Autodesk Fusion 360 part; units mm, degrees
note: some values were not read from the file. Chosen so that the rebuilt part matches the saved one: which bodies a step acts on; which face or edge a step refers to. Set by a fixed rule: which sketch regions a step uses.
(part 2 of 2)
sketch "hookLedge" plane through (0, 0, -2.5) normal (0, 0, -1) x (1, 0, 0)
  circle A0 centre (54.2689, -22.0155) radius 1.5
  circle A1 centre (176.25, -22.3937) radius 1.5
  circle A2 centre (176, -22.3937) radius 1.25
  circle A3 centre (146, -22.3937) radius 1.25
  circle A4 centre (176, -22.3937) radius 1.25
  circle A5 centre (146, -22.3937) radius 1.25
  circle A6 centre (4, -22.3937) radius 1.25
  circle A7 centre (54, -22.3937) radius 1.25
  circle A8 centre (4, -22.3937) radius 1.25
  circle A9 centre (54, -22.3937) radius 1.25
  line L0 (0, 0) -> (0, -40)
  line L1 (0, -40) -> (180, -40)
  line L2 (180, -40) -> (180, 0)
  line L3 (180, 0) -> (0, 0)
  line L4 (140.5, -33.5) -> (140.5, -27.75)
  line L5 (140.5, -27.75) -> (148, -27.75)
  line L6 (154.5, -33.5) -> (154.5, -24.7385)
  line L7 (154.5, -24.7385) -> (120, -24.7385)
  line L8 (120, -24.7385) -> (120, -27.7385)
  line L9 (120, -27.7385) -> (116.5, -27.7385)
  line L10 (116.5, -27.7385) -> (116.5, -24.7385)
  line L11 (116.5, -24.7385) -> (25.5, -24.7385)
  line L12 (25.5, -24.7385) -> (25.5, -33.5)
  line L13 (32, -27.75) -> (39.5, -27.75)
  line L14 (39.5, -27.75) -> (39.5, -33.5)
  line L15 (25.5, -33.5) -> (32, -33.5)
  line L16 (50.5, -33.5) -> (50.5, -36.5)
  line L17 (50.5, -36.5) -> (2, -36.5)
  line L18 (2, -36.5) -> (2, -3.5)
  line L19 (2, -3.5) -> (50.5, -3.5)
  line L20 (50.5, -3.5) -> (50.5, -6.5)
  line L21 (50.5, -6.5) -> (35.5, -6.5)
  line L22 (35.5, -15.2615) -> (116.5, -15.2615)
  line L23 (116.5, -15.2615) -> (116.5, -12.2615)
  line L24 (116.5, -12.2615) -> (120, -12.2615)
  line L25 (120, -12.2615) -> (120, -15.2615)
  line L26 (120, -15.2615) -> (144.5, -15.2615)
  line L27 (144.5, -6.5) -> (129.5, -6.5)
  line L28 (129.5, -6.5) -> (129.5, -3.5)
  line L29 (129.5, -3.5) -> (178, -3.5)
  line L30 (178, -3.5) -> (178, -36.5)
  line L31 (178, -36.5) -> (129.5, -36.5)
  line L32 (129.5, -36.5) -> (129.5, -33.5)
  line L33 (129.5, -33.5) -> (140.5, -33.5)
  line L34 (25.5, -24.4885) -> (174.5, -24.4885)
  line L35 (32.5, -15.5115) -> (25.5, -15.5115)
  line L36 (100, -24.4885) -> (100.0375, -15.4143)
  line L37 (90, -40) -> (90, 0)
  circle A10 centre (145.75, -22.3937) radius 1.5
  circle A11 centre (3.75, -22.3937) radius 1.5
  line L38 (144.5, -15.2615) -> (144.5, -6.5)
  line L39 (148, -27.75) -> (148, -33.5)
  line L40 (32, -33.5) -> (32, -27.75)
  circle A12 centre (145.75, -22.3937) radius 1.5
  circle A13 centre (54.2765, -21.879) radius 1.5
  line L41 (25.5, -15.5115) -> (25.5, -24.4885)
  line L42 (34.75, -17.7615) -> (32.5, -15.5115)
  line L43 (174.5, -24.4885) -> (174.5, -15.5115)
  line L44 (174.5, -15.5115) -> (167.5, -15.5115)
  line L45 (167.5, -15.5115) -> (165.25, -17.7615)
  line L46 (165.25, -17.7615) -> (144, -17.7615)
  line L47 (144, -17.7615) -> (144, -15.5115)
  line L48 (56, -15.5115) -> (56, -17.7615)
  line L49 (56, -17.7615) -> (34.75, -17.7615)
  line L50 (148, -33.5) -> (154.5, -33.5)
  line L51 (39.5, -33.5) -> (50.5, -33.5)
  line L52 (35.5, -6.5) -> (35.5, -15.2615)
  line L53 (144, -15.5115) -> (56, -15.5115)
  point P0 (176.25, -22.3937)
  dimension "d122" = 3
  dimension "d123" = 3
  constraint midpoint L34 L36.start
  constraint midpoint L1 L37.start
  constraint midpoint L3 L37.end
  constraint symmetric A0 L36 A10
  constraint symmetric A1 L37 A11
  constraint coincident A10.centre A12.centre
  constraint coincident P0 A1.centre
  measures "d122" diameter of A0
  measures "d123" diameter of A1
extrude "Extrude15" add sketch "hookLedge" along normal blind 1 contours A0 A7 A9 A13 | A0 A7 A9 A13 | A0 A7 A9 A13 | A0 A7 A9 A13 | A7 A9 A13 | A2 A4 | A1 | A3 A5 | A10 A12 | A6 A8 | A11 bodies 4 5 6
ref_plane "WorkPlane2" through (90, 20, 4.7) normal (0, 0, 1) x (1, 0, 0)
sketch "bladeCatch" plane through (75, 20, 4.7) normal (0, 0, 1) x (1, 0, 0)
  line L0 (99.75, 13.25) -> (99.75, -13.25)
  line L1 (67.45, -10) -> (72.75, -10)
  line L2 (72.75, -10) -> (72.75, 13.25)
  line L3 (72.75, 13.25) -> (69.75, 13.25)
  line L4 (69.75, 13.25) -> (69.75, -6)
  line L5 (69.75, -6) -> (67.45, -6)
  line L6 (99.75, -7.5) -> (67.45, -7.5)
  line L7 (67.45, -7.5) -> (67.45, 7.5)
  line L8 (67.45, 7.5) -> (99.75, 7.5)
  line L9 (99.75, 7.5) -> (99.75, -7.5)
  line L10 (72, -5.75) -> (72, -10)
  line L11 (72, -10) -> (67.45, -10)
  line L12 (72.75, -5.5) -> (67.45, -5.5)
  line L13 (67.45, -6) -> (67.45, -10)
  line L14 (67.45, -7.5) -> (67.4497, -7.75)
  line L15 (15, 20) -> (15, -20)
  line L16 (-42, -5.75) -> (-37.4497, -7.75)
  line L17 (-37.45, -6) -> (-37.45, -10)
  line L18 (-42, -10) -> (-37.45, -10)
  line L19 (-42, -5.75) -> (-42, -10)
  line L20 (83.6, 7.5) -> (83.6, -7.5707)
  line L21 (94.45, -5.5) -> (99.75, -5.5)
  line L22 (94.45, -10) -> (94.45, 13.25)
  line L23 (72, -5.75) -> (67.4497, -7.75)
  line L24 (73.5, 7.5) -> (73.5, -7.5)
  line L25 (93.7, 7.5) -> (93.7, -7.5)
  point P0 (99.75, 0)
  point P1 (99.75, -7.5)
  dimension "d163" = 7.5
  dimension "d166" = 15
  dimension "d167" = 0.75
  dimension "d168" = 1.75
  dimension "d171" = 0.25
  dimension "d296" = 0.25
  dimension "d337" = 0.75
  dimension "d338" = 0.75
  constraint midpoint L0 P0
  constraint coincident L0 P1
  constraint horizontal L6
  constraint vertical L7
  constraint horizontal L8
  constraint vertical L9
  constraint coincident P1 L6.start
  constraint perpendicular L7 L11
  constraint coincident L10.end L11.start
  constraint perpendicular L10 L11
  constraint coincident L1.start L11
  constraint coincident L2 L12.start
  constraint coincident L7 L12.end
  constraint perpendicular L7 L12
  constraint coincident L1.start L11.end
  constraint symmetric L1.start L15 L17.end
  constraint symmetric L5.end L15 L17.start
  constraint symmetric L10.start L15 L16.start
  constraint symmetric L10.end L15 L18.start
  constraint symmetric L14.end L15 L16.end
  constraint midpoint L8 L20.start
  constraint symmetric L1.end L20 L22.start
  constraint symmetric L2.end L20 L22.end
  constraint symmetric L12.start L20 L21.start
  constraint symmetric L12.end L20 L21.end
  constraint coincident L5.end L7
  constraint perpendicular L8 L20
  constraint coincident P1 L6
  constraint coincident L0 L8.end
  constraint coincident L8 L24.start
  constraint coincident L6 L24.end
  constraint perpendicular L6 L24
  constraint coincident L8 L25.start
  constraint coincident L6 L25.end
  constraint perpendicular L6 L25
  measures "d163" distance of P0 P1
  measures "d166" distance of P1 L8.end
  measures "d167" distance of L2 L10
  measures "d168" distance of L6 L10.start
  measures "d171" distance of L10.start L12
  measures "d296" distance of L6.end L14.end
  measures "d337" distance of L2 L24
  measures "d338" distance of L22 L25
extrude "Extrude18" add sketch "bladeCatch" along normal blind 1.3 separate body contours L1 L6 L10 L11 L13 L23 | L6 L10 L23 | L16 L17 L18 L19 makes body 7 at (144.1562, 10.8333, 4.7) makes body 8 at (34.5167, 12.1667, 4.7)
extrude "Extrude19" add 1 faces at (144.1562, 10.8333, 4.7) along direction (0, 0, -1) blind 0.7 on bodies 7 bodies 7 2
chamfer "Chamfer4" distance 0.7 angle 45 2 edges at (142.45, 11.1251, 6) (37.55, 11.1251, 6) on bodies 7 8
extrude "Extrude42" add 1 faces at (34.5167, 12.1667, 4.7) along direction (0, 0, -1) blind 0.7 on bodies 8 bodies 8 6 3
extrude "Extrude20" add sketch "bladeCatch" along normal blind 2 separate body contours L0 L8 L9 L21 L22 | L6 L8 L22 L25 | L6 L8 L20 L25 | L6 L8 L20 L24 | L2 L6 L8 L24 | L2 L4 L8 L12 | L4 L7 L8 L12 makes body 9
extrude "Extrude48" cut sketch "bladeCatch" along normal blind 0.35 contours L0 L8 L9 L21 L22 | L6 L8 L22 L25 | L2 L6 L8 L24 | L2 L4 L8 L12 | L4 L7 L8 L12 bodies 9
ref_plane "WorkPlane3" through (158.6, 20, 9.2) normal (0, 0, 1) x (1, 0, 0)
sketch "blade" plane through (0, 0, 9.2) normal (0, 0, 1) x (-1, 0, 0)
  line L0 (-174.75, -20) -> (-174.75, -7.5)
  line L1 (-174.75, -20) -> (-174.75, -32.5)
  line L2 (-174.75, -20) -> (0.25, -20)
  spline S0 degree 5 poles (0.25, -20) (-0.613, -21.2348) (-4.217, -23.503) (-15.2513, -26.3014) (-39.5964, -28.9809) (-80.2085, -31.0875) (-116.9511, -32.0515) (-145.5572, -32.4184) (-164.9632, -32.5) (-174.75, -32.5) knots 0 0 0 0 0 0 0.2 0.4 0.6 0.8 1 1 1 1 1 1
  line L3 (-154.0742, -32.5) -> (-195.4258, -32.5)
  line L4 (1.7905, -17.796) -> (-1.2905, -22.204)
  spline S1 degree 5 poles (0.25, -20) (-0.613, -18.7652) (-4.217, -16.497) (-15.2513, -13.6986) (-39.5964, -11.0191) (-80.2085, -8.9125) (-116.9511, -7.9485) (-145.5572, -7.5816) (-164.9632, -7.5) (-174.75, -7.5) knots 0 0 0 0 0 0 0.2 0.4 0.6 0.8 1 1 1 1 1 1
  line L5 (1.7905, -22.204) -> (-1.2905, -17.796)
  line L6 (-154.0742, -7.5) -> (-195.4258, -7.5)
  line L7 (-174.75, -27.5) -> (-142.45, -27.5)
  line L8 (-142.45, -27.5) -> (-142.45, -14.5)
  line L9 (-142.45, -14.5) -> (-147.75, -14.5)
  line L10 (-147.75, -14.5) -> (-147.75, -12.5)
  line L11 (-147.75, -12.5) -> (-169.45, -12.5)
  line L12 (-169.45, -12.5) -> (-169.45, -14.5)
  line L13 (-169.45, -14.5) -> (-174.75, -14.5)
  line L14 (-174.75, -14.5) -> (-174.75, -27.5)
  line L15 (-174.75, -14.5) -> (-174.75, -12.5)
  line L16 (-174.75, -12.5) -> (-174.75, -27.5)
  dimension "d178" = 12.5
  dimension "d179" = 12.5
  dimension "d180" = 175
  dimension "d307" = 15
  constraint midpoint L1.end L3
  constraint midpoint L2.end L4
  constraint symmetric L1.end L2 L0.end
  constraint symmetric S0.start L2 S1.start
  constraint symmetric L2 L3.start L6.start
  constraint symmetric L2 L3.end L6.end
  constraint symmetric L2 L4.start L5.start
  constraint symmetric L2 L4.end L5.end
  constraint coincident L13.end L14.start
  constraint perpendicular L13 L15
  constraint coincident L7.start L14.end
  constraint perpendicular L7 L16
  constraint midpoint L0.start L16
  constraint perpendicular L2 L16
  constraint perpendicular L1 L3
  constraint parallel L1 L16
  measures "d178" distance of L0.start L0.end
  measures "d179" distance of L0.start L1.end
  measures "d180" distance of L0.start L2.end
  measures "d307" distance of L15.end L7.start
extrude "Extrude21" add sketch "blade" against normal blind 2.5 bodies 9
extrude "Extrude22" add 1 faces at (139.2419, 23.4266, 9.2) along direction (0, 0, 1) blind 2.5 on bodies 9 bodies 9
fillet "Fillet1" radius 2.5 4 edges at (60.8718, 29.9001, 11.7) (60.8718, 10.0999, 11.7) (60.8718, 29.9001, 6.7) (60.8718, 10.0999, 6.7) on bodies 9
sketch "bladeSlide" plane through (0, 0, 11.7) normal (0, 0, 1) x (-1, 0, 0)
  line L0 (-174.75, -10) -> (-174.75, -30)
  line L1 (-148.5, -27.5) -> (-168.7, -27.5)
  line L2 (-168.7, -12.5) -> (-148.5, -12.5)
  line L3 (-174.75, -20) -> (-174.75, -17.5)
  line L4 (-174.75, -17.5) -> (-142.45, -17.5)
  line L5 (-142.45, -17.5) -> (-142.45, -22.5)
  line L6 (-142.45, -22.5) -> (-174.75, -22.5)
  line L7 (-174.75, -22.5) -> (-174.75, -17.5)
  line L8 (-175, -22.75) -> (-175, -17.25)
  line L9 (-175, -22.75) -> (-5, -22.75)
  line L10 (-5, -22.75) -> (-5, -17.25)
  line L11 (-5, -17.25) -> (-175, -17.25)
  line L12 (-180, -27.75) -> (0, -27.75)
  line L13 (0, -27.75) -> (0, -12.25)
  line L14 (0, -12.25) -> (-180, -12.25)
  line L15 (-180, -12.25) -> (-180, -27.75)
  spline S0 degree 3 poles (-3.932, -20) (-4.006, -20.0344) (-4.0803, -20.0681) (-5.0177, -20.486) (-5.9124, -20.8014) (-8.8794, -21.7323) (-10.9913, -22.2135) (-15.2343, -23.0595) (-17.369, -23.4153) (-22.9443, -24.247) (-26.394, -24.6645) (-33.3023, -25.4018) (-36.7614, -25.7195) (-47.1439, -26.5766) (-54.073, -27.0224) (-61.009, -27.4038) (-70.4768, -27.9244) (-79.9549, -28.3213) (-98.9091, -28.9731) (-108.3858, -29.2255) (-136.8174, -29.8197) (-155.7857, -30) (-174.75, -30) knots -17.152951 -17.152951 -17.152951 -17.152951 -17.128445 -17.128445 -16.844648 -16.844648 -16.195539 -16.195539 -15.546431 -15.546431 -14.504463 -14.504463 -13.462494 -13.462494 -11.378553 -11.378553 -11.378553 -8.533915 -8.533915 -5.689277 -5.689277 0 0 0 0
  line L16 (-180, 0) -> (-180, -40)
  spline S1 degree 3 poles (-174.75, -10) (-155.7857, -10) (-136.8174, -10.1803) (-108.3858, -10.7745) (-98.9091, -11.0269) (-79.9549, -11.6787) (-70.4768, -12.0756) (-61.009, -12.5962) (-54.073, -12.9776) (-47.1439, -13.4234) (-36.7614, -14.2805) (-33.3023, -14.5982) (-26.394, -15.3355) (-22.9443, -15.753) (-17.369, -16.5847) (-15.2343, -16.9405) (-10.9913, -17.7865) (-8.8794, -18.2677) (-5.9124, -19.1986) (-5.0177, -19.514) (-4.0803, -19.9319) (-4.006, -19.9656) (-3.932, -20) knots -17.412242 -17.412242 -17.412242 -17.412242 -11.722965 -11.722965 -8.878327 -8.878327 -6.033689 -6.033689 -6.033689 -3.949748 -3.949748 -2.907779 -2.907779 -1.865811 -1.865811 -1.216703 -1.216703 -0.567594 -0.567594 -0.283797 -0.283797 -0.259291 -0.259291 -0.259291 -0.259291
  line L17 (-148.5, -12.5) -> (-148.5, -27.5)
  line L18 (-168.7, -27.5) -> (-168.7, -12.5)
  line L19 (-142.45, -12.5) -> (-142.45, -27.5)
  line L20 (-174.75, -27.5) -> (-174.75, -12.5)
  point P0 (-174.75, -20)
  point P1 (-145.0002, -20)
  point P2 (-180, -20)
  point P3 (-180, -20)
  dimension "d207" = 2.5
  dimension "d208" = 5
  dimension "d209" = 5.5
  dimension "d210" = 0.25
  dimension "d211" = 0.25
  dimension "d212" = 170
  dimension "d214" = 5
  dimension "d215" = 5
  dimension "d216" = 5
  dimension "d343" = 5
  constraint coincident P0 L3.start
  constraint vertical L5
  constraint vertical L7
  constraint vertical L8
  constraint horizontal L12
  constraint vertical L13
  constraint horizontal L14
  constraint vertical L15
  constraint midpoint L15 P3
  constraint midpoint L16 P3
  constraint coincident P3 P2
  constraint perpendicular L5 L6
  constraint perpendicular L3 L4
  constraint perpendicular L8 L11
  constraint perpendicular L4 L5
  constraint coincident L5.end L19
  measures "d207" distance of P0 L3.end
  measures "d208" distance of L3.end L6.end
  measures "d209" distance of L8.start L8.end
  measures "d210" vertical distance of L6.end L8.start
  measures "d211" distance of L7 L8.start
  measures "d212" distance of L8.start L9.end
  measures "d214" distance of L8 L15
  measures "d215" distance of L10 L13
  measures "d216" distance of L9 L12
  measures "d343" distance of L11 L14
extrude "Extrude23" add sketch "bladeSlide" along normal blind 2 contours L0 L3 L4 L6 L7 L18 L20 | L4 L6 L17 L18 | L4 L5 L6 L17 L19 bodies 9
extrude "Extrude24" add sketch "bladeSlide" along normal blind 2 separate body contours L0 L8 L9 L11 L12 L14 L15 L16 L20 | L0 L2 L11 L14 S1 L17 L18 L20 | L2 L11 L17 L18 | L0 L1 L9 L12 S0 L17 L18 L20 | L1 L9 L17 L18 | L9 L10 L11 L12 L13 L14 S0 S1 | L10 S0 S1 makes body 10
sketch "boltHoles" plane through (0, 0, 13.7) normal (0, 0, 1) x (-1, 0, 0)
  line L0 (-5, -22.75) -> (-175, -22.75)
  line L1 (-175, -22.75) -> (-175, -17.25)
  line L2 (-175, -17.25) -> (-5, -17.25)
  line L3 (-5, -17.25) -> (-5, -22.75)
  line L4 (-180, -12.25) -> (-180, -27.75)
  line L5 (-180, -27.75) -> (0, -27.75)
  line L6 (0, -27.75) -> (0, -12.25)
  line L7 (0, -12.25) -> (-180, -12.25)
  line L8 (-125, -27.75) -> (-117.2, -27.75)
  line L9 (-117.2, -27.75) -> (-117.2, -40)
  line L10 (-117.2, -40) -> (-125, -40)
  line L11 (-125, -40) -> (-125, -27.75)
  line L12 (-117.2, -37.1) -> (-125, -37.1)
  line L13 (-180, -40) -> (0, -40)
  line L14 (0, 0) -> (-180, 0)
  circle A0 centre (-121.1, -37.1) radius 1.9
  circle A1 centre (-121.1, -37.1) radius 1.15
  line L15 (-180, 0) -> (-180, -40)
  line L16 (0, -40) -> (0, 0)
  line L17 (-117.2, -34.2) -> (-125, -34.2)
  line L18 (0, -20) -> (-180, -20)
  line L19 (-90, -40) -> (-90, 0)
  line L20 (-180, -40) -> (-176.1, -40)
  line L21 (-176.1, -40) -> (-176.1, -39.15)
  circle A2 centre (-176.1, -39.15) radius 1.15
  circle A3 centre (-176.1, -39.15) radius 1.9
  line L22 (-176.1, -39.15) -> (-180, -39.15)
  line L23 (-176.1, -39.15) -> (-172.2, -39.15)
  line L24 (-172.2, -39.15) -> (-172.2, -42.05)
  line L25 (-172.2, -39.15) -> (-172.2, -36.25)
  line L26 (-172.2, -36.25) -> (-180, -36.25)
  line L27 (-172.2, -42.05) -> (-180, -42.05)
  line L28 (-180, -42.05) -> (-180, -39.15)
  line L29 (-180, -39.15) -> (-180, -36.25)
  line L30 (-117.2, -12.25) -> (-117.2, 0)
  line L31 (-176.1, -0.85) -> (-172.2, -0.85)
  line L32 (-117.2, 0) -> (-125, 0)
  line L33 (-180, 0) -> (-176.1, 0)
  circle A4 centre (-176.1, -0.85) radius 1.9
  line L34 (-172.2, -3.75) -> (-180, -3.75)
  line L35 (-176.1, 0) -> (-176.1, -0.85)
  line L36 (-117.2, -5.8) -> (-125, -5.8)
  line L37 (-176.1, -0.85) -> (-180, -0.85)
  line L38 (-180, -0.85) -> (-180, -3.75)
  line L39 (-180, 2.05) -> (-180, -0.85)
  circle A5 centre (-121.1, -2.9) radius 1.9
  line L40 (-117.2, -2.9) -> (-125, -2.9)
  line L41 (-172.2, -0.85) -> (-172.2, 2.05)
  line L42 (-125, 0) -> (-125, -12.25)
  line L43 (-125, -12.25) -> (-117.2, -12.25)
  line L44 (-172.2, 2.05) -> (-180, 2.05)
  line L45 (-172.2, -0.85) -> (-172.2, -3.75)
  circle A6 centre (-121.1, -2.9) radius 1.15
  circle A7 centre (-176.1, -0.85) radius 1.15
  line L46 (-7.8, -39.15) -> (-7.8, -42.05)
  line L47 (-3.9, -0.85) -> (-7.8, -0.85)
  line L48 (0, -0.85) -> (0, -3.75)
  line L49 (0, -39.15) -> (0, -36.25)
  line L50 (0, -12.25) -> (0, -27.75)
  circle A8 centre (-58.9, -37.1) radius 1.9
  line L51 (0, 2.05) -> (0, -0.85)
  line L52 (-7.8, -42.05) -> (0, -42.05)
  line L53 (-5, -22.75) -> (-5, -17.25)
  line L54 (-3.9, -40) -> (-3.9, -39.15)
  line L55 (-7.8, -0.85) -> (-7.8, 2.05)
  circle A9 centre (-58.9, -2.9) radius 1.15
  line L56 (-3.9, -39.15) -> (-7.8, -39.15)
  line L57 (0, 0) -> (0, -40)
  line L58 (-62.8, -12.25) -> (-62.8, 0)
  line L59 (-7.8, -39.15) -> (-7.8, -36.25)
  line L60 (-7.8, -36.25) -> (0, -36.25)
  line L61 (-55, 0) -> (-55, -12.25)
  line L62 (-7.8, -3.75) -> (0, -3.75)
  line L63 (-62.8, -27.75) -> (-62.8, -40)
  line L64 (-7.8, 2.05) -> (0, 2.05)
  line L65 (-7.8, -0.85) -> (-7.8, -3.75)
  line L66 (-62.8, -5.8) -> (-55, -5.8)
  line L67 (-3.9, -39.15) -> (0, -39.15)
  line L68 (0, 0) -> (-3.9, 0)
  line L69 (-62.8, -34.2) -> (-55, -34.2)
  circle A10 centre (-3.9, -0.85) radius 1.9
  line L70 (0, -42.05) -> (0, -39.15)
  circle A11 centre (-3.9, -0.85) radius 1.15
  circle A12 centre (-3.9, -39.15) radius 1.9
  line L71 (-3.9, -0.85) -> (0, -0.85)
  line L72 (-55, -40) -> (-55, -27.75)
  line L73 (-55, -27.75) -> (-62.8, -27.75)
  circle A13 centre (-3.9, -39.15) radius 1.15
  line L74 (-62.8, -40) -> (-55, -40)
  circle A14 centre (-58.9, -37.1) radius 1.15
  line L75 (-62.8, -37.1) -> (-55, -37.1)
  line L76 (-62.8, 0) -> (-55, 0)
  circle A15 centre (-58.9, -2.9) radius 1.9
  line L77 (-3.9, 0) -> (-3.9, -0.85)
  line L78 (-55, -12.25) -> (-62.8, -12.25)
  line L79 (0, -40) -> (-3.9, -40)
  line L80 (-62.8, -2.9) -> (-55, -2.9)
  line L81 (-172.2, -36.25) -> (-172.2, -27.75)
  line L82 (-172.2, -27.75) -> (-180, -27.75)
  line L83 (-180, -36.25) -> (-180, -27.75)
  line L84 (-180, -36.25) -> (-180, -27.75)
  line L85 (-172.2, -3.75) -> (-172.2, -12.25)
  line L86 (-180, -3.75) -> (-180, -12.25)
  line L87 (-172.2, -12.25) -> (-180, -12.25)
  line L88 (-7.8, -36.25) -> (-7.8, -27.75)
  line L89 (0, -36.25) -> (0, -27.75)
  line L90 (-7.8, -27.75) -> (0, -27.75)
  line L91 (-7.8, -12.25) -> (0, -12.25)
  line L92 (0, -3.75) -> (0, -12.25)
  line L93 (-7.8, -3.75) -> (-7.8, -12.25)
  point P0 (-121.1, -37.1)
  point P1 (-180, -12.25)
  point P2 (-180, 0)
  point P3 (-121.1, -2.9)
  point P4 (-58.9, -2.9)
  point P5 (0, -12.25)
  point P6 (0, -20)
  point P7 (-58.9, -37.1)
  dimension "d227" = 2.9
  dimension "d228" = 7.8
  dimension "d229" = 3.8
  dimension "d230" = 2.3
  dimension "d232" = 55
  dimension "d249" = 2.9
  dimension "d326" = 3.9
  dimension "d328" = 2.3
  dimension "d329" = 3.8
  dimension "d330" = 3.9
  dimension "d331" = 3.9
  dimension "d332" = 2.9
  dimension "d333" = 2.9
  dimension "d334" = 0.85
  constraint horizontal L8
  constraint vertical L9
  constraint horizontal L10
  constraint vertical L11
  constraint coincident L5 L8.start
  constraint coincident L9 L12.start
  constraint coincident L11 L12.end
  constraint perpendicular L11 L12
  constraint midpoint L12 P0
  constraint coincident L10.end L13
  constraint coincident P0 A0.centre
  constraint concentric A0 A1
  constraint coincident L9 L17.start
  constraint coincident L11 L17.end
  constraint midpoint L16 P6
  constraint midpoint L15 L18.end
  constraint midpoint L13 L19.start
  constraint midpoint L14 L19.end
  constraint coincident L13.start L15.end
  constraint coincident L13 L20.end
  constraint perpendicular L15 L20
  constraint perpendicular L20 L21
  constraint coincident L21.end A2.centre
  constraint concentric A2 A3
  constraint perpendicular L21 L22
  constraint perpendicular L21 L23
  constraint perpendicular L23 L24
  constraint perpendicular L13 L25
  constraint coincident L15 L26.end
  constraint perpendicular L15 L26
  constraint perpendicular L24 L27
  constraint symmetric L4.end L18 P1
  constraint symmetric L8.start L18 L42.end
  constraint symmetric L8.end L18 L30.start
  constraint symmetric L9.end L18 L30.end
  constraint symmetric L10.end L18 L32.end
  constraint symmetric L12.start L18 L40.start
  constraint symmetric L12.end L18 L40.end
  constraint symmetric P0 L18 P3
  constraint symmetric L13.start L18 P2
  constraint symmetric A0 L18 A5
  constraint symmetric A1 L18 A6
  constraint symmetric L17.start L18 L36.start
  constraint symmetric L17.end L18 L36.end
  constraint symmetric L18 L13.start P2
  constraint symmetric L18 L20.end L33.end
  constraint symmetric L18 L21.end L31.start
  constraint symmetric L18 A2 A7
  constraint symmetric L18 A3 A4
  constraint symmetric L18 L22.end L37.end
  constraint symmetric L18 L23.end L31.end
  constraint symmetric L18 L24.end L41.end
  constraint symmetric L18 L25.end L34.start
  constraint symmetric L18 L26.end L34.end
  constraint symmetric L18 L27.end L39.start
  constraint symmetric L0.end L19 L0.start
  constraint symmetric L1.end L19 L2.end
  constraint symmetric P1 L19 L6.end
  constraint symmetric L4.end L19 L5.end
  constraint symmetric L8.start L19 L72.end
  constraint symmetric L8.end L19 L63.start
  constraint symmetric L9.end L19 L63.end
  constraint symmetric L10.end L19 L72.start
  constraint symmetric L12.start L19 L75.start
  constraint symmetric L12.end L19 L75.end
  constraint symmetric P0 L19 P7
  constraint symmetric L13.start L19 L13.end
  constraint symmetric P2 L19 L14.start
  constraint symmetric A0 L19 A8
  constraint symmetric A1 L19 A14
  constraint symmetric L17.start L19 L69.start
  constraint symmetric L17.end L19 L69.end
  constraint symmetric L18.end L19 P6
  constraint symmetric L19 L13.start L13.end
  constraint symmetric L19 L20.end L54.start
  constraint symmetric L19 L21.end L54.end
  constraint symmetric L19 A2 A13
  constraint symmetric L19 A3 A12
  constraint symmetric L19 L22.end L49.start
  constraint symmetric L19 L23.end L46.start
  constraint symmetric L19 L24.end L46.end
  constraint symmetric L19 L25.end L59.end
  constraint symmetric L19 L26.end L49.end
  constraint symmetric L19 L27.end L52.end
  constraint symmetric L19 L31.start L47.start
  constraint symmetric L19 L37.end L48.start
  constraint symmetric L19 L36.end L66.end
  constraint symmetric L19 L39.start L51.start
  constraint symmetric L19 L32.end L61.start
  constraint symmetric L19 P2 L14.start
  constraint symmetric L19 P1 P5
  constraint symmetric L19 L30.start L58.start
  constraint symmetric L19 L33.end L68.end
  constraint symmetric L19 L30.end L58.end
  constraint symmetric L19 L34.end L48.end
  constraint symmetric L19 L40.start L80.start
  constraint symmetric L19 L34.start L62.start
  constraint symmetric L19 L31.end L47.end
  constraint symmetric L19 L41.end L55.end
  constraint symmetric L19 L36.start L66.start
  constraint symmetric L19 L40.end L80.end
  constraint symmetric L19 P3 P4
  constraint symmetric L19 L42.end L61.end
  constraint symmetric L19 A4 A10
  constraint symmetric L19 A5 A15
  constraint symmetric L19 A6 A9
  constraint symmetric L19 A7 A11
  constraint coincident L5 L81.end
  constraint perpendicular L5 L81
  constraint coincident L4.end L5.start
  constraint symmetric L18 L81.end L85.end
  constraint symmetric L18 L4.end P1
  constraint symmetric L19 L81.end L88.end
  constraint symmetric L19 L4.end L5.end
  constraint symmetric L19 L85.end L91.start
  measures "d227" distance of L10 L12
  measures "d228" distance of L9 L11
  measures "d229" diameter of A0
  measures "d230" diameter of A1
  measures "d232" distance of L11 L15
  measures "d249" distance of L12 L17
  measures "d326" distance of L13.start L20.end
  measures "d328" diameter of A2
  measures "d329" diameter of A3
  measures "d330" distance of L21.end L22.end
  measures "d331" distance of L21.end L23.end
  measures "d332" distance of L23.end L24.end
  measures "d333" distance of L23.end L25.end
  measures "d334" distance of L13.start L22
sketch "boltAttachment" plane through (0, 0, 4) normal (0, 0, 1) x (-1, 0, 0)
  line L0 (-28, -6.5) -> (-28, -9)
  line L1 (-28, -9) -> (-32, -9)
  line L2 (-32, -9) -> (-32, -33.5)
  line L3 (-32, -33.5) -> (-35.5, -33.5)
  line L4 (-35.5, -33.5) -> (-35.5, -30.25)
  line L5 (-35.5, -30.25) -> (-39.5, -30.25)
  line L6 (-39.5, -30.25) -> (-39.5, -27.75)
  line L7 (-39.5, -27.75) -> (-35.5, -27.75)
  line L8 (-35.5, -27.75) -> (-35.5, -14.25)
  line L9 (-35.5, -14.25) -> (-54.5, -14.25)
  line L10 (-54.5, -14.25) -> (-54.5, -6.5)
  line L11 (-54.5, -6.5) -> (-28, -6.5)
  line L12 (-2, -2) -> (-2, -38)
  line L13 (-2, -38) -> (-24.5, -38)
  line L14 (-24.5, -38) -> (-24.5, -33.25)
  line L15 (-24.5, -33.25) -> (-25.5, -33.25)
  line L16 (-25.5, -33.25) -> (-25.5, -6.5)
  line L17 (-25.5, -6.5) -> (-24.5, -6.5)
  line L18 (-24.5, -6.5) -> (-24.5, -2)
  line L19 (-24.5, -2) -> (-2, -2)
  line L20 (-178, -38) -> (-178, -2)
  line L21 (-178, -2) -> (-155.5, -2)
  line L22 (-155.5, -2) -> (-155.5, -6.5)
  line L23 (-155.5, -6.5) -> (-154.5, -6.5)
  line L24 (-154.5, -6.5) -> (-154.5, -33.5)
  line L25 (-154.5, -33.5) -> (-155.5, -33.5)
  line L26 (-155.5, -33.5) -> (-155.5, -38)
  line L27 (-155.5, -38) -> (-178, -38)
  line L28 (-125.5, -6.5) -> (-125.5, -14.25)
  line L29 (-125.5, -14.25) -> (-144.5, -14.25)
  line L30 (-144.5, -14.25) -> (-144.5, -27.75)
  line L31 (-144.5, -27.75) -> (-140.5, -27.75)
  line L32 (-140.5, -27.75) -> (-140.5, -30.25)
  line L33 (-140.5, -30.25) -> (-144.5, -30.25)
  line L34 (-144.5, -30.25) -> (-144.5, -33.5)
  line L35 (-144.5, -33.5) -> (-148, -33.5)
  line L36 (-148, -33.5) -> (-148, -9)
  line L37 (-148, -9) -> (-152, -9)
  line L38 (-152, -9) -> (-152, -6.5)
  line L39 (-152, -6.5) -> (-125.5, -6.5)
  line L40 (-120, -27.7385) -> (-120, -12.2615)
  line L41 (-120, -12.2615) -> (-93.5, -12.2615)
  line L42 (-93.5, -12.2615) -> (-93.5, -27.7385)
  line L43 (-93.5, -27.7385) -> (-120, -27.7385)
  line L44 (0, -40) -> (0, 0)
  line L45 (0, 0) -> (-180, 0)
  line L46 (-180, 0) -> (-180, -40)
  line L47 (-180, -40) -> (0, -40)
  line L48 (-7.8, -42.05) -> (0, -42.05)
  line L49 (-7.8, -39.15) -> (-7.8, -42.05)
  line L50 (0, -42.05) -> (0, -39.15)
  line L51 (-7.8, -0.85) -> (-7.8, 2.05)
  line L52 (-7.8, 2.05) -> (0, 2.05)
  line L53 (0, 2.05) -> (0, -0.85)
  line L54 (-180, -42.05) -> (-180, -39.15)
  line L55 (-172.2, -42.05) -> (-180, -42.05)
  line L56 (-172.2, -39.15) -> (-172.2, -42.05)
  line L57 (-180, 2.05) -> (-180, -0.85)
  line L58 (-172.2, -0.85) -> (-172.2, 2.05)
  line L59 (-172.2, 2.05) -> (-180, 2.05)
sketch "springHolder" plane through (0, 0, 4) normal (0, 0, 1) x (-1, 0, 0)
  line L0 (-28, -6.5) -> (-28, -9)
  line L1 (-28, -9) -> (-32, -9)
  line L2 (-32, -9) -> (-32, -33.5)
  line L3 (-32, -33.5) -> (-35.5, -33.5)
  line L4 (-35.5, -33.5) -> (-35.5, -30.25)
  line L5 (-35.5, -30.25) -> (-39.5, -30.25)
  line L6 (-39.5, -30.25) -> (-39.5, -27.75)
  line L7 (-39.5, -27.75) -> (-35.5, -27.75)
  line L8 (-35.5, -27.75) -> (-35.5, -14.25)
  line L9 (-35.5, -14.25) -> (-54.5, -14.25)
  line L10 (-54.5, -14.25) -> (-54.5, -6.5)
  line L11 (-54.5, -6.5) -> (-28, -6.5)
  line L12 (-2, -2) -> (-2, -38)
  line L13 (-2, -38) -> (-24.5, -38)
  line L14 (-24.5, -38) -> (-24.5, -33.25)
  line L15 (-24.5, -33.25) -> (-25.5, -33.25)
  line L16 (-25.5, -33.25) -> (-25.5, -6.5)
  line L17 (-25.5, -6.5) -> (-24.5, -6.5)
  line L18 (-24.5, -6.5) -> (-24.5, -2)
  line L19 (-24.5, -2) -> (-2, -2)
  line L20 (-178, -38) -> (-178, -2)
  line L21 (-178, -2) -> (-155.5, -2)
  line L22 (-155.5, -2) -> (-155.5, -6.5)
  line L23 (-155.5, -6.5) -> (-154.5, -6.5)
  line L24 (-154.5, -6.5) -> (-154.5, -33.5)
  line L25 (-154.5, -33.5) -> (-155.5, -33.5)
  line L26 (-155.5, -33.5) -> (-155.5, -38)
  line L27 (-155.5, -38) -> (-178, -38)
  line L28 (-125.5, -6.5) -> (-125.5, -14.25)
  line L29 (-125.5, -14.25) -> (-144.5, -14.25)
  line L30 (-144.5, -14.25) -> (-144.5, -27.75)
  line L31 (-144.5, -27.75) -> (-140.5, -27.75)
  line L32 (-140.5, -27.75) -> (-140.5, -30.25)
  line L33 (-140.5, -30.25) -> (-144.5, -30.25)
  line L34 (-144.5, -30.25) -> (-144.5, -33.5)
  line L35 (-144.5, -33.5) -> (-148, -33.5)
  line L36 (-148, -33.5) -> (-148, -9)
  line L37 (-148, -9) -> (-152, -9)
  line L38 (-152, -9) -> (-152, -6.5)
  line L39 (-152, -6.5) -> (-125.5, -6.5)
  line L40 (-120, -27.7385) -> (-120, -12.2615)
  line L41 (-120, -12.2615) -> (-93.5, -12.2615)
  line L42 (-93.5, -12.2615) -> (-93.5, -27.7385)
  line L43 (-93.5, -27.7385) -> (-120, -27.7385)
  line L44 (0, -40) -> (0, 0)
  line L45 (0, 0) -> (-180, 0)
  line L46 (-180, 0) -> (-180, -40)
  line L47 (-180, -40) -> (0, -40)
  line L48 (-90, 0) -> (-41, 0)
  line L49 (-41, 0) -> (-90, 0)
  line L50 (-90, 0) -> (-90, -11.75)
  line L51 (-90, -11.75) -> (-41, -11.75)
  line L52 (-41, -11.75) -> (-41, 0)
  line L53 (-139, -11.75) -> (-139, 0)
  line L54 (-90, -11.75) -> (-139, -11.75)
  line L55 (-168.7, -12.5) -> (-148.5, -12.5)
  dimension "d317" = 49
  dimension "d325" = 0.75
  constraint midpoint L45 L48.start
  constraint coincident L45 L48.end
  constraint perpendicular L8 L48
  constraint horizontal L49
  constraint vertical L50
  constraint horizontal L51
  constraint vertical L52
  constraint symmetric L48.end L50 L53.end
  constraint symmetric L51.start L50 L54.start
  constraint symmetric L51.end L50 L53.start
  constraint coincident L48.start L49.end
  measures "d317" distance of L48.start L48.end
  measures "d325" distance of L54 L55
extrude "Extrude44" add sketch "springHolder" along normal blind 1 separate body contours L10 L11 L51 L52 | L10 L11 L45 L48 L49 L50 L51 L52 | L28 L39 L45 L50 L53 L54 | L28 L39 L53 L54 makes body 11
extrude "Extrude43" add sketch "boltAttachment" against normal blind 4 contours L47 L48 L49 L50 | L47 L54 L55 L56 | L45 L51 L52 L53 | L45 L57 L58 L59 bodies 1 11 4 5 6 7 8
extrude "Extrude25" add sketch "boltHoles" against normal blind 2 contours L5 L8 L9 L11 L17 | L5 L63 L69 L72 L73 | L5 L16 L57 L60 L88 L89 L90 | L7 L16 L57 L62 L91 L92 L93 | L9 L11 L12 A0 L17 | A8 L63 L69 L72 L75 | L9 L10 L11 L12 L13 A0 | L13 A8 L63 L72 L74 L75 | L16 L49 L56 L57 L59 L60 L67 A12 | L16 L47 L48 L57 L62 L65 A10 L71 | L7 L15 L34 L85 L86 L87 | L5 L15 L26 L81 L82 L83 L84 | L7 L58 L61 L66 L78 | L7 L30 L36 L42 L43 | L13 L16 L57 L67 L70 A12 L79 | L14 L16 L51 L57 L68 A10 L71 | L15 L31 A4 L34 L37 L38 L45 | L15 A3 L22 L23 L25 L26 L29 | L13 L20 A3 L24 L27 L28 | L13 A3 L23 L24 | L13 L46 L56 A12 | L13 L46 L52 L70 A12 L79 | L58 L61 L66 A15 L80 | L30 L36 A5 L40 L42 | L14 L58 L61 L76 A15 L80 | L14 L30 L32 A5 L40 L42 | L14 L47 L55 A10 | L14 L51 L55 L64 L68 A10 | L14 L15 L33 A4 L37 L39 | L13 L15 L20 A3 L22 L28 | L14 L31 A4 L41 | L14 L33 A4 L39 L41 L44 bodies 10
extrude "Extrude26" add sketch "boltHoles" against normal blind 9.7 contours L9 L11 L12 A0 L17 | A8 L63 L69 L72 L75 | L9 L10 L11 L12 L13 A0 | L13 A8 L63 L72 L74 L75 | L16 L49 L56 L57 L59 L60 L67 A12 | L16 L47 L48 L57 L62 L65 A10 L71 | L13 L16 L57 L67 L70 A12 L79 | L14 L16 L51 L57 L68 A10 L71 | L15 L31 A4 L34 L37 L38 L45 | L15 A3 L22 L23 L25 L26 L29 | L12 A0 A1 | L12 A0 A1 | A8 A14 L75 | A8 A14 L75 | L13 L20 A3 L24 L27 L28 | L13 A3 L23 L24 | L13 L46 L56 A12 | L13 L46 L52 L70 A12 L79 | L58 L61 L66 A15 L80 | L30 L36 A5 L40 L42 | L14 L58 L61 L76 A15 L80 | L14 L30 L32 A5 L40 L42 | L13 L67 A12 A13 L79 | L56 L67 A12 A13 | L14 L47 L55 A10 | L14 L51 L55 L64 L68 A10 | L14 L68 A10 A11 L71 | L47 A10 A11 L71 | L14 L15 L33 A4 L37 L39 | L13 L15 L20 A3 L22 L28 | L13 L20 A2 A3 | L13 A2 A3 L23 | L13 L56 A12 A13 | L13 A12 A13 L79 | L14 L47 A10 A11 | L14 L68 A10 A11 | L14 L31 A4 L41 | L14 L33 A4 L39 L41 L44 | L31 A4 L37 A7 | L14 L33 A4 L37 A7 | L13 L20 A2 A3 L22 | A2 A3 L22 L23 | A9 A15 L80 | A9 A15 L80 | A5 L40 A6 | A5 L40 A6 | L14 L31 A4 A7 | L14 L33 A4 A7 bodies 10
extrude "Extrude47" cut sketch "puller" along normal blind 5.4 contours L0 L2 L19 L41 L55 | L2 L10 L16 L17 L23 L24 L32 L33 L44 L45 | L0 L10 L41 L42 L44 L45 | L0 L3 L5 L19 L55 L56 | L0 L3 L10 L42 L45 L51 L56 | L10 L42 L43 L44 L45 L46 L47 L48 L52 | L10 L42 L43 L44 L45 | L10 L46 L49 L50 L51 L52 | L16 L30 L31 L32 L33 L34 L35 L36 L40 | L16 L30 L31 L32 L33 | L1 L16 L29 L30 L32 L33 | L1 L6 L16 L30 L33 L39 L54 | L1 L2 L18 L29 L53 | L16 L34 L37 L38 L39 L40 | L1 L6 L8 L18 L53 L54 | L58 L63 L64 L88 L90 | L58 L63 L64 L78 L88 L90 L91 L94 L99 | L63 L64 L84 L88 L90 L101 | L64 L70 L84 L86 L88 L90 L92 | L59 L63 L64 L68 L90 L95 L98 L105 L107 L108 | L64 L70 L87 L89 L94 L99 | L60 L84 L96 L101 L105 | L60 L75 L84 L86 L92 L96 | L59 L61 L62 L68 L69 L77 L95 L100 L106 | L59 L65 L68 L69 L81 L95 | L59 L61 L68 L69 L95 | L59 L65 L69 L74 L83 L95 L97 | L65 L81 L103 L105 L109 | L74 L77 L80 L95 L106 L111 | L65 L76 L83 L97 L103 L109 bodies 10
combine "Combine1" operation cut target body 10 tool bodies 11 keep tools
extrude "Extrude27" cut sketch "boltHoles" against normal blind 2 contours L12 A0 A1 | L12 A0 A1 | A8 A14 L75 | A8 A14 L75 | L13 L67 A12 A13 L79 | L56 L67 A12 A13 | L14 L68 A10 A11 L71 | L47 A10 A11 L71 | L13 L20 A2 A3 | L13 A2 A3 L23 | L13 L56 A12 A13 | L13 A12 A13 L79 | L14 L47 A10 A11 | L14 L68 A10 A11 | L31 A4 L37 A7 | L14 L33 A4 L37 A7 | L13 L20 A2 A3 L22 | A2 A3 L22 L23 | A9 A15 L80 | A9 A15 L80 | A5 L40 A6 | A5 L40 A6 | L14 L31 A4 A7 | L14 L33 A4 A7 bodies 10
extrude "Extrude28" cut sketch "boltHoles" against normal blind 30 contours L12 A1 | L12 A1 | A14 L75 | A14 L75 | L13 L54 L67 A13 L79 | L56 L67 A13 | L14 L68 A11 L71 L77 | L47 A11 L71 | L13 L20 A2 | L13 L21 A2 L23 | L13 L54 L56 A13 | L13 A13 L79 | L14 L47 A11 L77 | L14 L68 A11 | L14 L33 L35 L37 A7 | L31 L37 A7 | L13 L20 L21 A2 L22 | A2 L22 L23 | A9 L80 | A9 L80 | L40 A6 | L40 A6 | L14 L31 L35 A7 | L14 L33 A7 bodies 1 11
chamfer "Chamfer2" distance 0.35 angle 45 4 edges at (148.5, 20, 4.7) (142.45, 21, 5.05) (174.75, 21, 5.05) (168.7, 20, 4.7) on bodies 9
extrude "Extrude34" add sketch "slide" against normal blind 5.5 contours L4 L5 L21 L26 L48 L49 L55 L70 bodies 6
split "Split1" by plane through (90, 20, 2) normal (0, 0, 1) bodies 1 makes body 12 at (98.8333, 5.7836, 0) makes body 13 at (28.5, 14.2577, 0) makes body 14 at (69.192, 26.0527, 4) makes body 15 at (129.2962, 11.8698, 2.6667) makes body 16 at (53.9876, 9.7489, 3.3333)
combine "Combine2" operation add target body 14 tool bodies 13 1
combine "Combine3" operation add target body 12 tool bodies 15 16
sketch "Sketch5" plane through (0, 0, 4) normal (0, 0, 1) x (-1, 0, 0)
  line L0 (-77.8167, -43) -> (-151, -43)
  line L1 (-151, -43) -> (-151, 7)
  line L2 (-151, 7) -> (-77.8167, 7)
  line L3 (-77.8167, 7) -> (-77.8167, -43)
  circle A0 centre (-51.5, -9.5) radius 2.5
  circle A1 centre (-128.5, -9.5) radius 2.5
  constraint horizontal L0
  constraint vertical L1
  constraint horizontal L2
  constraint vertical L3
extrude "Extrude9" [suppressed]
extrude "Extrude10" [suppressed]
extrude "Extrude29" [suppressed]
equation "width = 40 mm" comment "The overall width of the design"
equation "height = 180 mm" comment "The overall height/length of the design"
equation "d3 = width"
equation "d4 = height"
equation "catchDistance = 32 mm" comment "The distance of the catch from the end"
equation "tolerance = 0.25 mm" comment "Tolerance"
equation "catchMargin = 6.5 mm" comment "The catch distance from the wall"
equation "catchTravel = 2 mm" comment "The distance that the catch travels"
equation "rotationSpringDiameter = 6 mm" comment "The diameterof the rotation spring"
equation "rotationSpringWire = 0.5 mm" comment "The size of the spring wire"
equation "d12 = catchMargin"
equation "d13 = catchMargin"
equation "d14 = tolerance"
equation "d15 = tolerance"
equation "d17 = tolerance"
equation "d18 = d21"
equation "rotationSpringLength = 19 mm" comment "The length of the rotation spring"
equation "d20 = rotationSpringLength"
equation "d21 = catchTravel + tolerance * 2 + rotationSpringWire * 2"
equation "d23 = d21 + d22 + tolerance"
equation "d24 = rotationSpringDiameter / 2"
equation "d25 = rotationSpringDiameter - rotationSpringWire * 2"
equation "d26 = rotationSpringDiameter / 2"
equation "floorWidth = 2 mm" comment "The minimal width of a wall"
equation "d29 = floorWidth"
equation "d30 = floorWidth * 2"
equation "d34 = floorWidth"
equation "d36 = catchLength"
equation "wallWidth = 2 mm" comment "The width of the outside walls"
equation "slideDistance = 20 mm" comment "The distance that the slider travels"
equation "d39 = wallWidth"
equation "d40 = wallWidth + pullerHookLength"
equation "d41 = wallWidth + pullerHookLength"
equation "d42 = tolerance"
equation "d43 = tolerance"
equation "d44 = tolerance"
equation "d45 = tolerance"
equation "d46 = tolerance"
equation "d48 = d47"
equation "d49 = 5 mm + slideDistance"
equation "d50 = pullerLength"
equation "d51 = d49"
equation "d52 = slideDistance + tolerance"
equation "d53 = slideDistance + tolerance"
equation "d54 = slideDistance + tolerance"
equation "pullerLength = 3 mm" comment "The length of the back puller bar"
equation "d56 = pullerLength + tolerance * 2 + wallWidth"
equation "catchLength = 3 mm" comment "The length/width of the catch"
equation "d60 = slideDistance + tolerance * 2 + catchLength"
equation "d63 = tolerance"
equation "d64 = tolerance"
equation "d65 = tolerance"
equation "d66 = tolerance + slideDistance"
equation "d69 = catchTravel + tolerance"
equation "d70 = -floorWidth"
equation "d74 = tolerance"
equation "d75 = -floorWidth"
equation "d77 = 2 * floorWidth + floorTolerance"
equation "d79 = -floorWidth"
equation "floorTolerance = 0.7 mm" comment "The tolerance to remove from a part to get a flush depth fit"
equation "catchHookWidth = 2 mm" comment "The width of the hook that keeps the catch in place"
equation "catchHookLength = 4 mm" comment "The length of th ehook that keeps the catch in palce"
equation "d88 = catchHookLength"
equation "d89 = catchHookWidth"
equation "d90 = catchHookLength"
equation "d91 = catchHookWidth + tolerance * 2"
equation "d92 = tolerance"
equation "d94 = catchHookLength"
equation "d95 = catchHookWidth"
equation "d96 = tolerance"
equation "d97 = catchHookWidth + tolerance * 2"
equation "d98 = d21"
equation "d99 = -floorWidth"
equation "springLength = 27 mm" comment "The length of the spring (under slighty tension)"
equation "springInnerDiameter = 3 mm" comment "The inner diameter of the spring"
equation "d107 = springInnerDiameter"
equation "d109 = springInnerDiameter"
equation "springHookDist = 2 mm" comment "The distance of the slot of the hook"
equation "springHookSlot = 0.5 mm" comment "The size of the hook slot"
equation "springHookLedge = 1 mm" comment "The size of the ledge of the hook"
equation "d114 = springHookDist"
equation "d120 = springHookSlot"
equation "d122 = springInnerDiameter"
equation "d123 = springInnerDiameter"
equation "d124 = springHookLedge"
equation "d126 = springHookSlot / 2"
equation "d127 = springHookSlot / 2"
equation "d128 = springInnerDiameter - springHookSlot"
equation "d129 = springInnerDiameter - springHookSlot"
equation "pullerHookLength = 1.5 mm" comment "The length of the puller hook"
equation "pullerHookWidth = 2 mm" comment "The width of the puller hook"
equation "slideHookLength = 3 mm" comment "The length of the slide hook"
equation "slideHookWidth = 3 mm" comment "The width of the slide hook"
equation "d136 = pullerHookWidth"
equation "d137 = pullerHookLength"
equation "d138 = pullerHookWidth + tolerance * 2"
equation "d139 = pullerHookLength"
equation "d140 = slideDistance"
equation "d141 = pullerHookWidth"
equation "d142 = pullerHookLength"
equation "d143 = pullerHookWidth + tolerance * 2"
equation "d144 = pullerHookLength"
equation "d145 = slideDistance"
equation "d146 = slideHookWidth"
equation "d147 = slideHookLength"
equation "d148 = slideHookWidth"
equation "d149 = slideHookLength"
equation "d150 = slideHookWidth + tolerance * 2"
equation "d151 = slideHookLength"
equation "d152 = pullerLength + tolerance"
equation "d153 = slideDistance + pullerLength"
equation "d154 = slideHookWidth + tolerance * 2"
equation "d155 = slideHookLength"
equation "slideCatchTolerance = 0.5 mm" comment "The distance at which the catch should release before the slide finished"
equation "d157 = 5 mm + rotationSpringLength"
equation "d158 = floorWidth - floorTolerance"
equation "additionalCatchFLoorTolerance = 0.25 mm" comment "Additional spacing for the catch"
equation "bladeHeight = 5 mm" comment "The height of the blade"
equation "d162 = floorTolerance"
equation "d163 = bladeCatchWidth / 2"
equation "bladeWidth = 25 mm" comment "The width of the blade"
equation "d166 = bladeCatchWidth"
equation "d167 = tolerance * 3"
equation "d168 = catchTravel - tolerance"
equation "bladeCatchWidth = 15 mm" comment "The width of the blade's part that interfaces with the catch"
equation "d171 = tolerance"
equation "d172 = floorWidth - floorTolerance"
equation "d174 = floorTolerance"
equation "d176 = floorWidth"
equation "d178 = bladeWidth / 2"
equation "d179 = bladeWidth / 2"
equation "d180 = height - wallWidth - pullerLength"
equation "d181 = bladeHeight / 2"
equation "d182 = -bladeHeight / 2"
equation "d184 = bladeHeight / 2"
equation "d205 = bladeHeight / 2"
equation "bladeSlideWidth = 5 mm" comment "The width of the slide area of the blade"
equation "d207 = bladeSlideWidth / 2"
equation "d208 = bladeSlideWidth"
equation "d209 = bladeSlideWidth + tolerance * 2"
equation "d210 = tolerance"
equation "d211 = tolerance"
equation "d212 = height - pullerLength * 2 - wallWidth * 2"
equation "d214 = wallWidth + pullerLength"
equation "d215 = pullerLength + wallWidth"
equation "d216 = bladeSlideWidth"
equation "d218 = floorWidth"
equation "d220 = wallWidth"
equation "boltDiameter = 2.3 mm" comment "The thread width"
equation "boltLength = 20 mm" comment "The total length of the bolt"
equation "boltHeadDiameter = 3.8 mm" comment "The diameter of the head"
equation "boltHeadLength = 2 mm" comment "The length of the head of the bolt"
equation "boltSpacing = 1 mm" comment "The wall width around bolts around bolts"
equation "d227 = boltHeadDiameter / 2 + boltSpacing"
equation "d228 = boltSpacing * 4 + boltHeadDiameter"
equation "d229 = boltHeadDiameter"
equation "d230 = boltDiameter"
equation "boltDistance = 55 mm" comment "The distance of the bolt from the back"
equation "d232 = boltDistance"
equation "d249 = boltHeadDiameter / 2 + boltSpacing"
equation "d253 = -floorWidth"
equation "d255 = -( floorTolerance + floorWidth * 2 + bladeHeight )"
equation "d257 = -boltHeadLength"
equation "d259 = wallWidth + pullerLength + tolerance"
equation "d264 = -floorTolerance"
equation "d266 = floorTolerance"
equation "d269 = -floorTolerance"
equation "d275 = -( floorWidth + springHookDist + springHookSlot + springHookLedge )"
equation "d277 = ( height - slideDistance ) / 2 - ( wallWidth + pullerLength + tolerance * 2 )"
equation "d279 = floorWidth"
equation "d281 = -floorWidth"
equation "d283 = -floorTolerance"
equation "d287 = floorTolerance"
equation "d288 = -floorTolerance"
equation "d290 = -floorWidth"
equation "d292 = -floorTolerance"
equation "d294 = 2 * floorWidth"
equation "d296 = tolerance"
equation "d297 = floorTolerance"
equation "preStretch = 5 mm" comment "The pre stretch distance to put on the spring in idle state"
equation "d302 = catchTravel"
equation "d303 = catchDistance"
equation "d304 = catchDistance - slideDistance + slideCatchTolerance"
equation "d305 = springInnerDiameter / 2 + wallWidth + tolerance"
equation "d306 = springLength - springInnerDiameter / 2 + preStretch"
equation "d307 = bladeCatchWidth"
equation "d315 = -floorWidth * 2"
equation "d317 = height / 2 - catchDistance - catchHookLength * 1.5 - catchLength"
equation "d319 = floorWidth / 2"
equation "d321 = floorTolerance / 2"
equation "d323 = -floorTolerance / 2"
equation "d325 = tolerance * 3"
equation "d326 = boltSpacing * 2 + boltHeadDiameter / 2"
equation "d328 = boltDiameter"
equation "d329 = boltHeadDiameter"
equation "d330 = boltSpacing * 2 + boltHeadDiameter / 2"
equation "d331 = boltSpacing * 2 + boltHeadDiameter / 2"
equation "d332 = boltSpacing + boltHeadDiameter / 2"
equation "d333 = boltSpacing + boltHeadDiameter / 2"
equation "d334 = wallWidth - boltDiameter / 2"
equation "d335 = floorWidth * 2 + floorTolerance * 2"
equation "d337 = tolerance * 3"
equation "d338 = tolerance * 3"
equation "d339 = floorTolerance / 2"
equation "d341 = floorTolerance / 2"
equation "d342 = floorTolerance"
equation "d343 = bladeSlideWidth"
named bodies: "base", "catch", "puller", "slide", "blade", "bladeRail", "catch2", "puller2", "springHolder", "bladeRail (1)", "base bottom", "base (2)", "base top", "base (4)", "base (5)"
